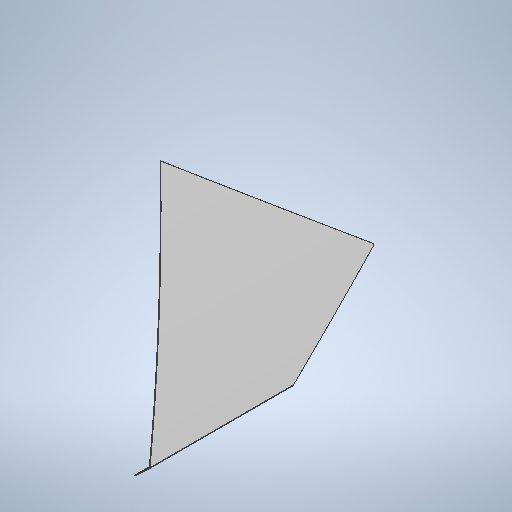
# Autodesk Inventor part: MSC 027.2 sheet board withers 4
Saved by Autodesk Inventor 2025 (Build 290162010, 162A)
## iProperties
Created: 2024-04-18
Part Number: MSC 027.2 sheet board withers 4
Material: AISI304
Document SubType Name: Sheet Metal
Designer: admin
Stock Number: МОО 027 лист левый-правый борт морда 1
Mass: 48027.3 g
Surface Area: 40202.8 cm^2
Volume: 6003.41 cm^3
Density: 8 g/cm^3
Sheet Metal Rule: Default_mm
Sheet Metal Width: 980,000 mm
Sheet Metal Length: 1322,653 mm
Sheet Metal Area: 1296200,418 mm^2
Appearance: Default
Flat Pattern Width: 98 cm
Flat Pattern Length: 132.265 cm
Flat Pattern Area: 12962 cm^2
Author: admin
Autodesk Inventor part; units mm, degrees
ref_plane "YZ Plane" through (0, 0, 0) normal (1, 0, 0) x (0, 1, 0)
ref_plane "XZ Plane" through (0, 0, 0) normal (0, 1, 0) x (-1, 0, 0)
ref_plane "XY Plane" through (0, 0, 0) normal (0, 0, 1) x (1, 0, 0)
sketch "Sketch1" plane through (0, 0, 0) normal (0, 0, 1) x (1, 0, 0)
  line L0 (-750, 0) -> (750, 0) construction
  line L1 (750, 0) -> (750, -2700) construction
  line L2 (750, -2700) -> (-750, -2700) construction
  line L3 (-750, -2700) -> (-750, 0) construction
  line L4 (800, 50) -> (-800, 50) construction
  line L5 (-800, 50) -> (-800, -2750) construction
  line L6 (-800, -2750) -> (800, -2750) construction
  line L7 (800, -2750) -> (800, 50) construction
  line L8 (-850, 100) -> (850, 100) construction
  line L9 (850, 100) -> (850, -2800) construction
  line L10 (850, -2800) -> (-850, -2800) construction
  line L11 (-850, -2800) -> (-850, 100) construction
  line L12 (-750, -2100) -> (750, -2100) construction
  line L13 (115.485997, -2697.8227) -> (682.456682, -2163.637569) construction
  arc A0 (750, -2100) -> (750.178737, -2098.125829) centre (-10250, -1050) ccw construction
  arc A1 (748.630029, -2101.290751) -> (750.178737, -2098.125829) centre (745.201281, -2097.651564) ccw
  arc A2 (110, -2700) -> (115.485997, -2697.8227) centre (110, -2692) ccw construction
  line L14 (-293.758559, -1127.507225) -> (682.456682, -2163.637569) construction
  arc A3 (750, 0) -> (0, 50) centre (0, -5600) ccw construction
  line L15 (0, 100) -> (0, 50) construction
  line L16 (0, -2700) -> (0, -1371.672536) construction
  line L17 (0, 1373.54809) -> (0, 0) construction
  line L18 (682.456682, -2163.637569) -> (748.630029, -2101.290751)
  arc A4 (750.178737, -2098.125829) -> (768.550013, -216.9) centre (-10250, -1050) ccw
  line L19 (748.630029, -2101.290751) -> (750, -2100) construction
  line L20 (768.550013, -216.9) -> (750, 0) construction
  point P0 (0, 0)
  point P1 (0, -2750)
  dimension "d130" = 1500
  dimension "d131" = 2700
  dimension "d132" = 2100
  dimension "d133" = 5
  dimension "d134" = 8
  dimension "d135" = 50
  dimension "d136" = 50
  dimension "d137" = 110
  dimension "d138" = 92.8
  dimension "d139" = 216.9
  measures "d130" distance of L0.start L0.end
  measures "d131" distance of L0.end L2.start
  measures "d132" distance between parallel lines of L12 L0
  measures "d133" radius of A1
  measures "d134" radius of A2
  measures "d135" distance between parallel lines of L4 L8
  measures "d136" distance between parallel lines of L0 L4
  measures "d137" distance from line of L16 A2.centre
  measures "d138" distance of L12.end L14.end
  measures "d139" vertical distance of L20.start L0.end
contour flange "Contour Flange2" sketch "Sketch1" thickness 3 bend radius 3 width 980 along (0, 0, 1) mid plane no both sides no wall seen from (715.543355, -2132.46416, 0) lies toward (0.6857497, -0.7278375, 0) curves L18 A1 A4
bend "Bend2"
corner "Corner2"
sketch "Sketch5" plane through (0, 0, 0) normal (1, 0, 0) x (0, 1, 0)
  line L0 (-2165.821082, 0) -> (-2165.821082, 980)
  line L1 (-2165.821082, 0) -> (-216.673819, 0)
  line L2 (-216.673819, 980) -> (-2165.821082, 980)
  line L3 (-872.673819, 980) -> (-1694.991458, 0)
  line L4 (-1704.991458, 0) -> (-2165.821082, 386.681968)
  line L5 (-216.673819, 0) -> (-216.673819, 980)
  point P0 (0, 0)
  dimension "d149" = 40
  dimension "d150" = 656
  dimension "d151" = 10
  constraints: 8 end point, 4 point on line, 2 horizontal, 1 perpendicular
  measures "d149" angle of L4 L1
  measures "d150" distance of L2.start L3.start
  measures "d151" distance of L3.end L4.start
extrude "Extrusion3" cut sketch "Sketch5" along normal through all both and the other way through all contours L0 L4 L1 | L3 L2 L5 L1
sketch "Sketch7" plane through (748.630029, -2101.290751, 980) normal (-0.6857497, 0.7278375, 0) x (0.7278375, 0.6857497, 0)
  line L0 (-54.728857, 87.67202) -> (-54.728857, 350.599522) construction
  line L1 (-54.728857, 350.599522) -> (-30.737155, 350.599522) construction
  line L2 (-30.737155, 350.599522) -> (-30.737155, 87.67202) construction
  line L3 (-30.737155, 87.67202) -> (-54.728857, 87.67202) construction
  point P0 (896.078441, 980)
  constraints: 2 other
mark "Mark4"
equation "\"d36\" = Thickness"
equation "\"d37\" = BendReliefWidth"
equation "\"d38\" = BendReliefDepth"
equation "\"d39\" = MinimumRemnant"
equation "\"d40\" = TransitionRadius"
equation "\"d42\" = BendRadius"
equation "\"d44\" = CornerReliefSize"
equation "\"d45\" = GapSize"
equation "\"d46\" = JacobiRadiusSize"
equation "\"BendRadius\" = Thickness"
equation "\"BendReliefWidth\" = Thickness"
equation "\"BendReliefDepth\" = 0.5 * Thickness"
equation "\"CornerReliefSize\" = 4 * Thickness"
equation "\"MinimumRemnant\" = 2 * Thickness"
equation "\"TransitionRadius\" = BendRadius"
equation "\"JacobiRadiusSize\" = BendRadius"
equation "\"GapSize\" = Thickness"
equation "\"Thickness\" = 3"
body "Solid3"
